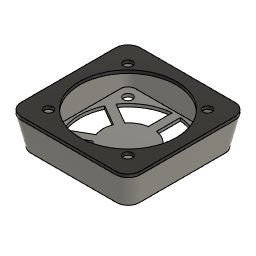
Fan Template - Bullseye (Autodesk Fusion 360 design; units mm, degrees)
Autodesk Fusion 360 part; units mm, degrees
sketch "Base Master" plane through (0, 0, 0) normal (0, 0, 1) x (1, 0, 0)
  circle A0 centre (0, 0) radius 19.5
  line L0 (16, -16) -> (-16, -16) construction
  line L1 (-16, -16) -> (-16, 16) construction
  line L2 (-16, 16) -> (16, 16) construction
  line L3 (16, 16) -> (16, -16) construction
  line L4 (16, -16) -> (-16, 16) construction
  line L5 (-16, -16) -> (16, 16) construction
  circle A1 centre (-16, 16) radius 1.8
  circle A2 centre (16, 16) radius 1.8
  circle A3 centre (16, -16) radius 1.8
  circle A4 centre (-16, -16) radius 1.8
  line L6 (17.25, -20.25) -> (-17.25, -20.25)
  line L7 (-20.25, -17.25) -> (-20.25, 17.25)
  line L8 (-17.25, 20.25) -> (17.25, 20.25)
  line L9 (20.25, 17.25) -> (20.25, -17.25)
  line L10 (20.25, -20.25) -> (-20.25, 20.25) construction
  line L11 (-20.25, -20.25) -> (20.25, 20.25) construction
  arc A5 (-17.25, 20.25) -> (-20.25, 17.25) centre (-17.25, 17.25) ccw
  arc A6 (20.25, 17.25) -> (17.25, 20.25) centre (17.25, 17.25) ccw
  arc A7 (17.25, -20.25) -> (20.25, -17.25) centre (17.25, -17.25) ccw
  arc A8 (-20.25, -17.25) -> (-17.25, -20.25) centre (-17.25, -17.25) ccw
  line L12 (-21.85, -17.25) -> (-21.85, 17.25)
  arc A9 (-17.25, 21.85) -> (-21.85, 17.25) centre (-17.25, 17.25) ccw
  line L13 (-17.25, 21.85) -> (17.25, 21.85)
  arc A10 (21.85, 17.25) -> (17.25, 21.85) centre (17.25, 17.25) ccw
  line L14 (21.85, 17.25) -> (21.85, -17.25)
  arc A11 (17.25, -21.85) -> (21.85, -17.25) centre (17.25, -17.25) ccw
  line L15 (17.25, -21.85) -> (-17.25, -21.85)
  arc A12 (-21.85, -17.25) -> (-17.25, -21.85) centre (-17.25, -17.25) ccw
  dimension "d10" = 39
  dimension "d11" = 32
  dimension "d12" = 32
  dimension "d13" = 3.6
  dimension "d14" = 3.6
  dimension "d15" = 3.6
  dimension "d16" = 3.6
  dimension "d18" = 40.5
  dimension "d19" = 40.5
  dimension "d20" = 3
  dimension "d21" = 3
  dimension "d22" = 3
  dimension "d23" = 3
  constraint coincident A0.centre origin
  constraint horizontal L0
  constraint perpendicular L0 L1
  constraint parallel L0 L2
  constraint parallel L1 L3
  constraint coincident L4 A0.centre
  constraint coincident L5 A0.centre
  constraint coincident L1.end L2.start
  constraint coincident L2.end L3.start
  constraint coincident L0.start L3.end
  constraint coincident L0.end L1.start
  constraint horizontal L6
  constraint perpendicular L6 L7
  constraint parallel L6 L8
  constraint parallel L7 L9
  constraint coincident L10 A0.centre
  constraint coincident L11 A0.centre
  constraint coincident L10.end L7
  constraint coincident L10.end L8
  constraint tangent L7 A5
  constraint tangent L8 A5
  constraint coincident L11.end L8
  constraint coincident L11.end L9
  constraint tangent L8 A6
  constraint tangent L9 A6
  constraint coincident L10.start L9
  constraint coincident L10.start L6
  constraint tangent L9 A7
  constraint tangent L6 A7
  constraint coincident L11.start L7
  constraint coincident L11.start L6
  constraint tangent L7 A8
  constraint tangent L6 A8
  measures "d10" diameter of A0
  measures "d11" distance of L1.end L2.end
  measures "d12" distance of L0.end L1.end
  measures "d13" diameter of A1
  measures "d14" diameter of A2
  measures "d15" diameter of A4
  measures "d16" diameter of A3
  measures "d18" distance of L10.end L11.end
  measures "d19" distance of L11.start L10.end
  measures "d20" radius of A5
  measures "d21" radius of A6
  measures "d22" radius of A7
  measures "d23" radius of A8
sketch "Base Loft" plane through (0, 0, 0) normal (0, 0, 1) x (1, 0, 0)
  arc A0 (21.85, 17.25) -> (17.25, 21.85) centre (17.25, 17.25) ccw
  line L0 (21.85, 17.25) -> (21.85, -17.25)
  arc A1 (17.25, -21.85) -> (21.85, -17.25) centre (17.25, -17.25) ccw
  line L1 (17.25, -21.85) -> (-17.25, -21.85)
  arc A2 (-21.85, -17.25) -> (-17.25, -21.85) centre (-17.25, -17.25) ccw
  line L2 (-21.85, -17.25) -> (-21.85, 17.25)
  arc A3 (-17.25, 21.85) -> (-21.85, 17.25) centre (-17.25, 17.25) ccw
  line L3 (-17.25, 21.85) -> (17.25, 21.85)
  arc A4 (20.25, 17.25) -> (17.25, 20.25) centre (17.25, 17.25) ccw
  line L4 (20.25, 17.25) -> (20.25, -17.25)
  arc A5 (17.25, -20.25) -> (20.25, -17.25) centre (17.25, -17.25) ccw
  line L5 (17.25, -20.25) -> (-17.25, -20.25)
  arc A6 (-20.25, -17.25) -> (-17.25, -20.25) centre (-17.25, -17.25) ccw
  line L6 (-20.25, -17.25) -> (-20.25, 17.25)
  arc A7 (-17.25, 20.25) -> (-20.25, 17.25) centre (-17.25, 17.25) ccw
  line L7 (-17.25, 20.25) -> (17.25, 20.25)
ref_plane "WorkPlane1" through (0, 0, 11.7) normal (0, 0, 1) x (1, 0, 0)
sketch "Top Loft" plane through (0, 0, 11.7) normal (0, 0, 1) x (1, 0, 0)
  line L0 (19, -24) -> (-19, -24)
  line L1 (-24, -19) -> (-24, 19)
  line L2 (-19, 24) -> (19, 24)
  line L3 (24, 19) -> (24, -19)
  line L4 (24, -24) -> (-24, 24) construction
  line L5 (-24, -24) -> (24, 24) construction
  arc A0 (-19, 24) -> (-24, 19) centre (-19, 19) ccw
  arc A1 (24, 19) -> (19, 24) centre (19, 19) ccw
  arc A2 (-24, -19) -> (-19, -24) centre (-19, -19) ccw
  arc A3 (19, -24) -> (24, -19) centre (19, -19) ccw
  line L6 (-19, 22.4) -> (19, 22.4)
  arc A4 (22.4, 19) -> (19, 22.4) centre (19, 19) ccw
  line L7 (22.4, 19) -> (22.4, -19)
  arc A5 (19, -22.4) -> (22.4, -19) centre (19, -19) ccw
  line L8 (19, -22.4) -> (-19, -22.4)
  arc A6 (-22.4, -19) -> (-19, -22.4) centre (-19, -19) ccw
  line L9 (-22.4, -19) -> (-22.4, 19)
  arc A7 (-19, 22.4) -> (-22.4, 19) centre (-19, 19) ccw
  dimension "d27" = 48
  dimension "d28" = 48
  dimension "d29" = 5
  dimension "d30" = 5
  dimension "d31" = 5
  dimension "d32" = 5
  dimension "d33" = 1.6
  constraint horizontal L0
  constraint perpendicular L0 L1
  constraint parallel L0 L2
  constraint parallel L1 L3
  constraint coincident L4 origin
  constraint coincident L5 origin
  constraint coincident L4.end L1
  constraint coincident L4.end L2
  constraint tangent L1 A0
  constraint tangent L2 A0
  constraint coincident L5.end L2
  constraint coincident L5.end L3
  constraint tangent L2 A1
  constraint tangent L3 A1
  constraint coincident L5.start L1
  constraint coincident L5.start L0
  constraint tangent L1 A2
  constraint tangent L0 A2
  constraint coincident L4.start L3
  constraint coincident L4.start L0
  constraint tangent L3 A3
  constraint tangent L0 A3
  measures "d27" distance of L4.end L5.end
  measures "d28" distance of L5.start L4.end
  measures "d29" radius of A0
  measures "d30" radius of A1
  measures "d31" radius of A2
  measures "d32" radius of A3
loft "Loft1" add profiles "Base Loft", "Top Loft" section 1 section 2 contours L0 L1 L2 L3 A0 A1 A2 A3 | L6 A4 L7 A5 L8 A6 L9 A7 makes body 1 in component "Fan Cage"
loft "Loft2" cut profiles "Top Loft", "Base Loft" section 1 contours L6 A4 L7 A5 L8 A6 L9 A7 section 2 contours A4 L4 A5 L5 A6 L6 A7 L7 bodies 1 in component "Fan Cage"
extrude "Extrude1" add sketch "Base Master" along normal blind 1.2 contours L6 L7 L8 L9 A5 A6 A7 A8 | L12 A9 L13 A10 L14 A11 L15 A12 bodies 1 in component "Fan Cage"
sketch "Sketch4" plane through (0, 0, 0) normal (0, 0, 1) x (1, 0, 0)
  circle A0 centre (0, 0) radius 10
  line L0 (0, 0) -> (0, 20) construction
  line L1 (1.6679, 9.8599) -> (1.6679, 19.4285)
  line L2 (-1.6679, 9.8599) -> (-1.6679, 19.4285)
  circle A1 centre (0, 0) radius 19.5
  line L3 (-7.705, 6.3744) -> (-15.9917, 11.1587)
  line L4 (-9.3729, 3.4855) -> (-17.6596, 8.2698)
  line L5 (-9.3729, -3.4855) -> (-17.6596, -8.2698)
  line L6 (-7.705, -6.3744) -> (-15.9917, -11.1587)
  line L7 (-1.6679, -9.8599) -> (-1.6679, -19.4285)
  line L8 (1.6679, -9.8599) -> (1.6679, -19.4285)
  line L9 (7.705, -6.3744) -> (15.9917, -11.1587)
  line L10 (9.3729, -3.4855) -> (17.6596, -8.2698)
  line L11 (9.3729, 3.4855) -> (17.6596, 8.2698)
  line L12 (7.705, 6.3744) -> (15.9917, 11.1587)
  dimension "d38" = 20
  dimension "d41" = 360
  constraint coincident A0.centre L0.start
  constraint vertical L0
  constraint parallel L0 L1
  constraint coincident A0 L1.start
  constraint symmetric L0 L1.end L2.end
  constraint symmetric L0 L1.start L2.start
  constraint coincident L2.end A1
  measures "d38" diameter of A0
extrude "Extrude2" add sketch "Sketch4" along normal up to surface (1.2 mm away) contours A0 | A0 A1 L11 L12 | A0 A1 L9 L10 | A0 L1 L2 A1 | A0 A1 L7 L8 | A0 A1 L3 L4 | A0 A1 L5 L6 bodies 1 in component "Fan Cage"
sketch "Sketch5" plane through (0, 0, 11.7) normal (0, 0, 1) x (1, 0, 0)
  circle A0 centre (-16, 16) radius 1.8
  circle A1 centre (16, 16) radius 1.8
  circle A2 centre (16, -16) radius 1.8
  circle A3 centre (-16, -16) radius 1.8
  spline S0 degree 3 poles (-24, -19) (-24, -20.325) (-23.4473, -21.6414) (-22.5015, -22.5693) (-21.5784, -23.4748) (-20.293, -24) (-19, -24) (-6.4171, -24) (6.4171, -24) (19, -24) (20.325, -24) (21.6414, -23.4473) (22.5693, -22.5015) (23.4748, -21.5784) (24, -20.293) (24, -19) (24, -6.4171) (24, 6.4171) (24, 19) (24, 20.325) (23.4473, 21.6414) (22.5015, 22.5693) (21.5784, 23.4748) (20.293, 24) (19, 24) (6.4171, 24) (-6.4171, 24) (-19, 24) (-20.325, 24) (-21.6414, 23.4473) (-22.5693, 22.5015) (-23.4748, 21.5784) (-24, 20.293) (-24, 19) (-24, 6.4171) (-24, -6.4171) (-24, -19) knots 0 0 0 0 0.021791 0.021791 0.021791 0.043057 0.043057 0.043057 0.25 0.25 0.25 0.271791 0.271791 0.271791 0.293057 0.293057 0.293057 0.5 0.5 0.5 0.521791 0.521791 0.521791 0.543057 0.543057 0.543057 0.75 0.75 0.75 0.771791 0.771791 0.771791 0.793057 0.793057 0.793057 1 1 1 1
  circle A4 centre (0, 0) radius 19.5
extrude "Extrude1'" add sketch "Sketch5" along normal blind 1.2 separate body makes body 2 in component "TPU Gasket"
component "Fan Cage" placed x (1, 0, 0) y (0, 1, 0) z (0, 0, 1) at (0, 0, 0)
component "TPU Gasket" placed x (1, 0, 0) y (0, 1, 0) z (0, 0, 1) at (0, 0, 0)
equation "fan_dia = 40 mm" comment "Diameter of the fan itself"
equation "hole_dia = fan_dia - 1 mm" comment "Actual size of the fan hole"
equation "screw_hole_dia = 3.6 mm" comment "Screw hole size"
equation "screw_hole_spacing = 32 mm" comment "Space between screws"
equation "fillet_fan = 3 mm" comment "Radius of fan edge fillet"
equation "fillet_wide = 5 mm" comment "Radius of large edge fillet"
equation "inside_margin = 1 mm" comment "Space around fan inside cage"
equation "fan_thickness = 10 mm" comment "Thickness of fan"
equation "wide_edge = fan_dia + 8 mm" comment "Distance between widest edges"
equation "d10 = hole_dia"
equation "d11 = screw_hole_spacing"
equation "d12 = screw_hole_spacing"
equation "d13 = screw_hole_dia"
equation "d14 = d13"
equation "d15 = d13"
equation "d16 = d13"
equation "narrow_edge = fan_dia + 0.5 mm" comment "Distance between shortest edges"
equation "d18 = narrow_edge"
equation "d19 = narrow_edge"
equation "d20 = fillet_fan"
equation "d21 = fillet_fan"
equation "d22 = fillet_fan"
equation "d23 = fillet_fan"
equation "wall_thickness = 1.6 mm"
equation "d25 = -wall_thickness"
equation "d26 = fan_thickness + face_thickness + 0.5 mm"
equation "d27 = wide_edge"
equation "d28 = wide_edge"
equation "d29 = fillet_wide"
equation "d30 = fillet_wide"
equation "d31 = fillet_wide"
equation "d32 = fillet_wide"
equation "d33 = wall_thickness"
equation "face_thickness = 1.2 mm" comment "Thickness of fan face"
equation "d35 = face_thickness"
equation "motor_dia = 20 mm" comment "Area in center covered by fan motor"
equation "d38 = motor_dia"
